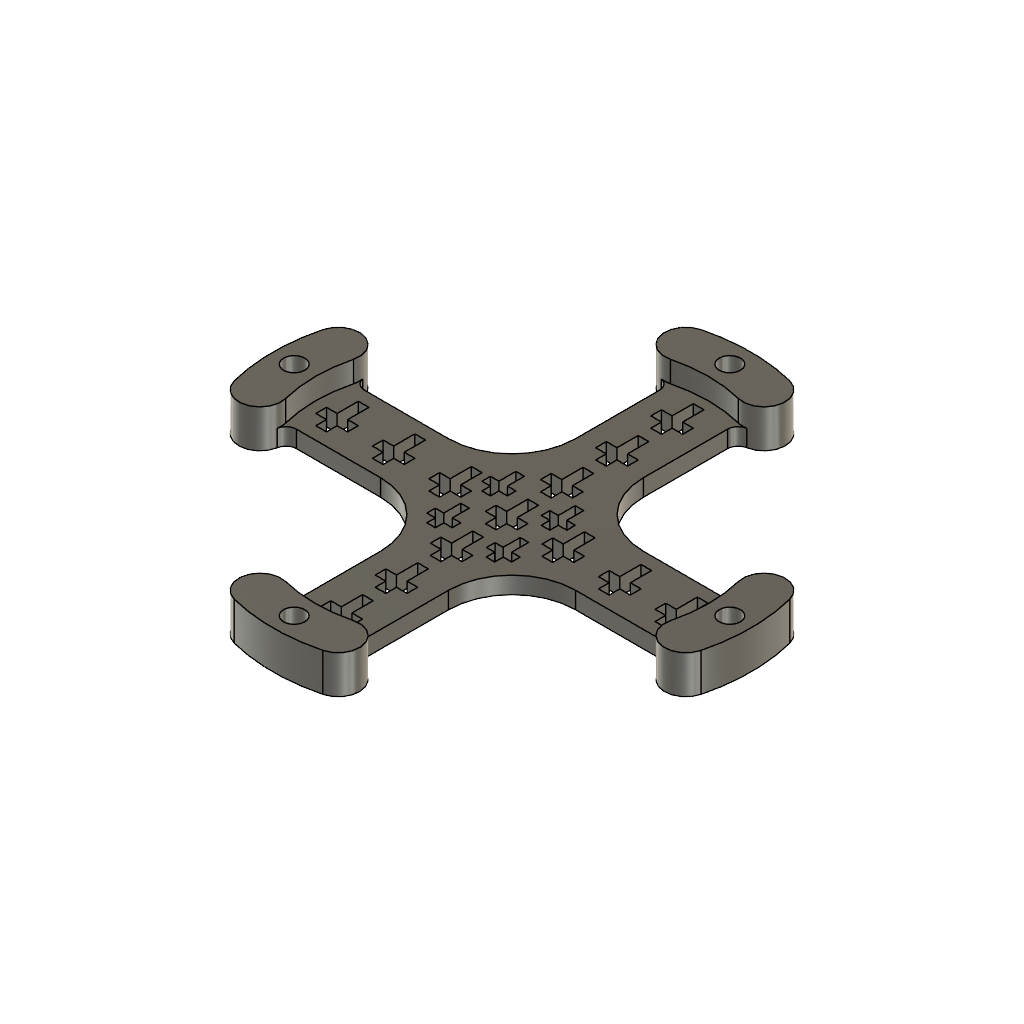
LR cross plus grill (Autodesk Fusion 360 design; units mm, degrees)
Autodesk Fusion 360 part; units mm, degrees
note: some values were not read from the file. Set by a fixed rule: which sketch regions a step uses.
(part 1 of 2)
sketch "Sketch1" plane through (0, 0, 0) normal (0, 0, 1) x (1, 0, 0)
  circle A0 centre (0, 0) radius 41.875
  line L0 (0, 41.875) -> (0, 45.375)
  line L1 (0, 45.375) -> (-8, 45.375)
  line L2 (0, 45.375) -> (8, 45.375)
  line L3 (0, 45.375) -> (0, 46.375)
  arc A1 (8, 45.375) -> (-8, 45.375) centre (0, 13.875) ccw
  arc A2 (10.4615, 55.0673) -> (-10.4615, 55.0673) centre (0, 13.875) ccw
  line L4 (-10.4615, 55.0673) -> (-8, 45.375)
  circle A3 centre (-9.2308, 50.2212) radius 5
  line L5 (0, 45.375) -> (0, 0)
  line L6 (-8, 45.375) -> (-8, 0)
  circle A4 centre (9.2308, 50.2212) radius 5
  line L7 (8, 45.375) -> (8, 0)
  line L8 (-45.375, 8) -> (0, 8)
  line L9 (-45.375, -8) -> (0, -8)
  circle A5 centre (-50.2212, -9.2308) radius 5
  arc A6 (-45.375, 8) -> (-45.375, -8) centre (-13.875, 0) ccw
  circle A7 centre (-50.2212, 9.2308) radius 5
  arc A8 (-55.0673, 10.4615) -> (-55.0673, -10.4615) centre (-13.875, 0) ccw
  line L10 (-8, -45.375) -> (-8, 0)
  line L11 (8, -45.375) -> (8, 0)
  circle A9 centre (9.2308, -50.2212) radius 5
  arc A10 (-8, -45.375) -> (8, -45.375) centre (0, -13.875) ccw
  circle A11 centre (-9.2308, -50.2212) radius 5
  arc A12 (-10.4615, -55.0673) -> (10.4615, -55.0673) centre (0, -13.875) ccw
  line L12 (45.375, -8) -> (0, -8)
  line L13 (45.375, 8) -> (0, 8)
  circle A13 centre (50.2212, 9.2308) radius 5
  arc A14 (45.375, -8) -> (45.375, 8) centre (13.875, 0) ccw
  circle A15 centre (50.2212, -9.2308) radius 5
  arc A16 (55.0673, -10.4615) -> (55.0673, 10.4615) centre (13.875, 0) ccw
  circle A17 centre (23, 23) radius 15
  circle A18 centre (-23, 23) radius 15
  circle A19 centre (-23, -23) radius 15
  circle A20 centre (23, -23) radius 15
  line L14 (0, 46.375) -> (0, 56.375)
  circle A21 centre (0, 51.375) radius 2.5
  circle A22 centre (-51.375, 0) radius 2.5
  circle A23 centre (0, -51.375) radius 2.5
  circle A24 centre (51.375, 0) radius 2.5
  arc A25 (-8, 42.8293) -> (-10.0769, 45.2933) centre (-10.5, 42.8293) ccw
  arc A26 (10.0769, 45.2933) -> (8, 42.8293) centre (10.5, 42.8293) ccw
  arc A27 (-42.8293, -8) -> (-45.2933, -10.0769) centre (-42.8293, -10.5) ccw
  arc A28 (-45.2933, 10.0769) -> (-42.8293, 8) centre (-42.8293, 10.5) ccw
  arc A29 (8, -42.8293) -> (10.0769, -45.2933) centre (10.5, -42.8293) ccw
  arc A30 (-10.0769, -45.2933) -> (-8, -42.8293) centre (-10.5, -42.8293) ccw
  arc A31 (42.8293, 8) -> (45.2933, 10.0769) centre (42.8293, 10.5) ccw
  arc A32 (45.2933, -10.0769) -> (42.8293, -8) centre (42.8293, -10.5) ccw
  dimension "d1" = 83.75
  dimension "d2" = 3.5
  dimension "d4" = 8
  dimension "d5" = 8
  dimension "d6" = 1
  dimension "d7" = 10
  dimension "d8" = 8
  dimension "d12" = 30
  dimension "d14" = 360
  dimension "d19" = 5
  dimension "d21" = 360
  dimension "d22" = 5
  dimension "d24" = 360
  constraint coincident A0.centre L5.end
  constraint coincident A0 L0.start
  constraint vertical L0
  constraint perpendicular L1 L3
  constraint coincident L3.end A1
  constraint midpoint L4 A3.centre
  constraint coincident A2.end A3
  constraint perpendicular L2 L5
  constraint symmetric A3 L5 A4
  constraint symmetric L5 L1.end L2.end
  constraint symmetric L5 L6.end L7.end
  constraint tangent L7 A17
  constraint tangent L13 A17
  constraint midpoint A2 L14.end
  constraint parallel L3 L14
  constraint midpoint L14 A21.centre
  constraint tangent A3 A25
  constraint tangent L6 A25
  constraint coincident A3 A25.end
  constraint coincident L6 A25.start
  constraint symmetric L5 A25.end A26.start
  constraint symmetric L5 A25 A26
  constraint symmetric L5 A25.start A26.end
  measures "d1" diameter of A0
  measures "d2" distance of L0.start L0.end
  measures "d4" distance of L0.end L1.end
  measures "d5" distance of L0.end L2.end
  measures "d6" distance of L0.end L3.end
  measures "d12" diameter of A17
  measures "d19" diameter of A21
  measures "d22" diameter of A25
extrude "Extrude1" add sketch "Sketch1" along normal blind 4 contours A0 L7 L11 L12 L13 | A0 L12 L13 A14 | L13 A13 A31 | L7 L13 A17 | L12 A15 A32 | L11 L12 A20 | A0 L5 L7 L13 | L6 L7 L8 L9 L10 L11 L12 L13 | A0 L9 L10 L11 L12 | A0 L0 L2 L5 L7 | A0 L5 L6 L8 | A0 L10 L11 A10 | A0 L0 L1 L5 L6 | A4 L7 A26 | L6 L8 A18 | A0 L6 L8 L9 L10 | L11 A9 A29 | L9 L10 A19 | L2 L3 A1 | L1 L3 A1 | L10 A11 A30 | A3 L6 A25 | A0 L8 L9 A6 | L8 A7 A28 | L9 A5 A27
extrude "Extrude2" add sketch "Sketch1" along normal blind 9 contours A13 | A13 A14 A15 A16 | A15 | A1 A2 A4 L14 A21 | A4 | A9 | A9 A10 A11 A12 | A1 A2 A3 L14 A21 | L4 A3 | L4 A3 | A11 | A5 A6 A7 A8 | A7 | A5
sketch "Sketch2" plane through (0, 0, 0) normal (0, 0, -1) x (1, 0, 0)
  circle A0 centre (0, 51.375) radius 2.5
  circle A1 centre (-51.375, 0) radius 2.5
  circle A2 centre (51.375, 0) radius 2.5
  circle A3 centre (0, -51.375) radius 2.5
  arc A4 (45.2933, -10.0769) -> (55.0673, -10.4615) centre (50.2212, -9.2308) ccw
  arc A5 (55.0673, -10.4615) -> (55.0673, 10.4615) centre (13.875, 0) ccw
  arc A6 (55.0673, 10.4615) -> (45.2933, 10.0769) centre (50.2212, 9.2308) ccw
  arc A7 (42.8293, 8) -> (45.2933, 10.0769) centre (42.8293, 10.5) ccw
  line L0 (42.8293, 8) -> (23, 8)
  arc A8 (8, 23) -> (23, 8) centre (23, 23) ccw
  line L1 (8, 23) -> (8, 42.8293)
  arc A9 (10.0769, 45.2933) -> (8, 42.8293) centre (10.5, 42.8293) ccw
  arc A10 (10.0769, 45.2933) -> (10.4615, 55.0673) centre (9.2308, 50.2212) ccw
  arc A11 (10.4615, 55.0673) -> (-10.4615, 55.0673) centre (0, 13.875) ccw
  arc A12 (-10.4615, 55.0673) -> (-10.0769, 45.2933) centre (-9.2308, 50.2212) ccw
  arc A13 (-8, 42.8293) -> (-10.0769, 45.2933) centre (-10.5, 42.8293) ccw
  line L2 (-8, 42.8293) -> (-8, 23)
  arc A14 (-23, 8) -> (-8, 23) centre (-23, 23) ccw
  line L3 (-23, 8) -> (-42.8293, 8)
  arc A15 (-45.2933, 10.0769) -> (-42.8293, 8) centre (-42.8293, 10.5) ccw
  arc A16 (-45.2933, 10.0769) -> (-55.0673, 10.4615) centre (-50.2212, 9.2308) ccw
  arc A17 (-55.0673, 10.4615) -> (-55.0673, -10.4615) centre (-13.875, 0) ccw
  arc A18 (-55.0673, -10.4615) -> (-45.2933, -10.0769) centre (-50.2212, -9.2308) ccw
  arc A19 (-42.8293, -8) -> (-45.2933, -10.0769) centre (-42.8293, -10.5) ccw
  line L4 (-42.8293, -8) -> (-23, -8)
  arc A20 (-8, -23) -> (-23, -8) centre (-23, -23) ccw
  line L5 (-8, -23) -> (-8, -42.8293)
  arc A21 (-10.0769, -45.2933) -> (-8, -42.8293) centre (-10.5, -42.8293) ccw
  arc A22 (-10.0769, -45.2933) -> (-10.4615, -55.0673) centre (-9.2308, -50.2212) ccw
  arc A23 (-10.4615, -55.0673) -> (10.4615, -55.0673) centre (0, -13.875) ccw
  arc A24 (10.4615, -55.0673) -> (10.0769, -45.2933) centre (9.2308, -50.2212) ccw
  arc A25 (8, -42.8293) -> (10.0769, -45.2933) centre (10.5, -42.8293) ccw
  line L6 (8, -42.8293) -> (8, -23)
  arc A26 (23, -8) -> (8, -23) centre (23, -23) ccw
  line L7 (23, -8) -> (42.8293, -8)
  arc A27 (45.2933, -10.0769) -> (42.8293, -8) centre (42.8293, -10.5) ccw
  line L8 (0, 0) -> (0, 5)
  line L9 (0, 5) -> (-1.25, 5)
  line L10 (-1.25, 5) -> (1.25, 5)
  line L11 (1.25, 5) -> (1.25, -5)
  line L12 (1.25, -5) -> (-1.25, -5)
  line L13 (-1.25, -5) -> (-1.25, 5)
  line L14 (-1.25, 5) -> (-1.25, 2.5)
  line L15 (-1.25, 2.5) -> (-3.75, 2.5)
  line L16 (-3.75, 2.5) -> (3.75, 2.5)
  line L17 (3.75, 2.5) -> (3.75, 0)
  line L18 (3.75, 0) -> (-3.75, 0)
  line L19 (-3.75, 0) -> (-3.75, 2.5)
  arc A28 (-8, -45.375) -> (8, -45.375) centre (0, -13.875) ccw
  arc A29 (-45.375, 8) -> (-45.375, -8) centre (-13.875, 0) ccw
  arc A30 (8, 45.375) -> (-8, 45.375) centre (0, 13.875) ccw
  arc A31 (45.375, -8) -> (45.375, 8) centre (13.875, 0) ccw
  line L20 (-38.75, -34) -> (-38.75, -44)
  line L21 (-41.25, -34) -> (-38.75, -34)
  line L22 (-41.25, -36.5) -> (-43.75, -36.5)
  line L23 (-41.25, -34) -> (-41.25, -36.5)
  line L24 (-43.75, -36.5) -> (-36.25, -36.5)
  line L25 (-40, -34) -> (-41.25, -34)
  line L26 (-40, -39) -> (-40, -34)
  line L27 (-41.25, -44) -> (-41.25, -34)
  line L28 (-43.75, -39) -> (-43.75, -36.5)
  line L29 (-38.75, -44) -> (-41.25, -44)
  line L30 (-36.25, -36.5) -> (-36.25, -39)
  line L31 (-36.25, -39) -> (-43.75, -39)
  line L32 (-25.4167, -34) -> (-25.4167, -44)
  line L33 (-27.9167, -34) -> (-25.4167, -34)
  line L34 (-27.9167, -36.5) -> (-30.4167, -36.5)
  line L35 (-27.9167, -34) -> (-27.9167, -36.5)
  line L36 (-30.4167, -36.5) -> (-22.9167, -36.5)
  line L37 (-26.6667, -34) -> (-27.9167, -34)
  line L38 (-26.6667, -39) -> (-26.6667, -34)
  line L39 (-27.9167, -44) -> (-27.9167, -34)
  line L40 (-30.4167, -39) -> (-30.4167, -36.5)
  line L41 (-25.4167, -44) -> (-27.9167, -44)
  line L42 (-22.9167, -36.5) -> (-22.9167, -39)
  line L43 (-22.9167, -39) -> (-30.4167, -39)
  line L44 (-12.0833, -34) -> (-12.0833, -44)
  line L45 (-14.5833, -34) -> (-12.0833, -34)
  line L46 (-14.5833, -36.5) -> (-17.0833, -36.5)
  line L47 (-14.5833, -34) -> (-14.5833, -36.5)
  line L48 (-17.0833, -36.5) -> (-9.5833, -36.5)
  line L49 (-13.3333, -34) -> (-14.5833, -34)
  line L50 (-13.3333, -39) -> (-13.3333, -34)
  line L51 (-14.5833, -44) -> (-14.5833, -34)
  line L52 (-17.0833, -39) -> (-17.0833, -36.5)
  line L53 (-12.0833, -44) -> (-14.5833, -44)
  line L54 (-9.5833, -36.5) -> (-9.5833, -39)
  line L55 (-9.5833, -39) -> (-17.0833, -39)
  line L56 (1.25, -34) -> (1.25, -44)
  line L57 (-1.25, -34) -> (1.25, -34)
  line L58 (-1.25, -36.5) -> (-3.75, -36.5)
  line L59 (-1.25, -34) -> (-1.25, -36.5)
  line L60 (-3.75, -36.5) -> (3.75, -36.5)
  line L61 (0, -34) -> (-1.25, -34)
  line L62 (0, -39) -> (0, -34)
  line L63 (-1.25, -44) -> (-1.25, -34)
  line L64 (-3.75, -39) -> (-3.75, -36.5)
  line L65 (1.25, -44) -> (-1.25, -44)
  line L66 (3.75, -36.5) -> (3.75, -39)
  line L67 (3.75, -39) -> (-3.75, -39)
  line L68 (14.5833, -34) -> (14.5833, -44)
  line L69 (12.0833, -34) -> (14.5833, -34)
  line L70 (12.0833, -36.5) -> (9.5833, -36.5)
  line L71 (12.0833, -34) -> (12.0833, -36.5)
  line L72 (9.5833, -36.5) -> (17.0833, -36.5)
  line L73 (13.3333, -34) -> (12.0833, -34)
  line L74 (13.3333, -39) -> (13.3333, -34)
  line L75 (12.0833, -44) -> (12.0833, -34)
  line L76 (9.5833, -39) -> (9.5833, -36.5)
  line L77 (14.5833, -44) -> (12.0833, -44)
  line L78 (17.0833, -36.5) -> (17.0833, -39)
  line L79 (17.0833, -39) -> (9.5833, -39)
  line L80 (27.9167, -34) -> (27.9167, -44)
  line L81 (25.4167, -34) -> (27.9167, -34)
  line L82 (25.4167, -36.5) -> (22.9167, -36.5)
  line L83 (25.4167, -34) -> (25.4167, -36.5)
  line L84 (22.9167, -36.5) -> (30.4167, -36.5)
  line L85 (26.6667, -34) -> (25.4167, -34)
  line L86 (26.6667, -39) -> (26.6667, -34)
  line L87 (25.4167, -44) -> (25.4167, -34)
  line L88 (22.9167, -39) -> (22.9167, -36.5)
  line L89 (27.9167, -44) -> (25.4167, -44)
  line L90 (30.4167, -36.5) -> (30.4167, -39)
  line L91 (30.4167, -39) -> (22.9167, -39)
  line L92 (41.25, -34) -> (41.25, -44)
  line L93 (38.75, -34) -> (41.25, -34)
  line L94 (38.75, -36.5) -> (36.25, -36.5)
  line L95 (38.75, -34) -> (38.75, -36.5)
  line L96 (36.25, -36.5) -> (43.75, -36.5)
  line L97 (40, -34) -> (38.75, -34)
  line L98 (40, -39) -> (40, -34)
  line L99 (38.75, -44) -> (38.75, -34)
  line L100 (36.25, -39) -> (36.25, -36.5)
  line L101 (41.25, -44) -> (38.75, -44)
  line L102 (43.75, -36.5) -> (43.75, -39)
  line L103 (43.75, -39) -> (36.25, -39)
  line L104 (-38.75, -21) -> (-38.75, -31)
  line L105 (-41.25, -21) -> (-38.75, -21)
  line L106 (-41.25, -23.5) -> (-43.75, -23.5)
  line L107 (-41.25, -21) -> (-41.25, -23.5)
  line L108 (-43.75, -23.5) -> (-36.25, -23.5)
  line L109 (-40, -21) -> (-41.25, -21)
  line L110 (-40, -26) -> (-40, -21)
  line L111 (-41.25, -31) -> (-41.25, -21)
  line L112 (-43.75, -26) -> (-43.75, -23.5)
  line L113 (-38.75, -31) -> (-41.25, -31)
  line L114 (-36.25, -23.5) -> (-36.25, -26)
  line L115 (-36.25, -26) -> (-43.75, -26)
  line L116 (-25.4167, -21) -> (-25.4167, -31)
  line L117 (-27.9167, -21) -> (-25.4167, -21)
  line L118 (-27.9167, -23.5) -> (-30.4167, -23.5)
  line L119 (-27.9167, -21) -> (-27.9167, -23.5)
  line L120 (-30.4167, -23.5) -> (-22.9167, -23.5)
  line L121 (-26.6667, -21) -> (-27.9167, -21)
  line L122 (-26.6667, -26) -> (-26.6667, -21)
  line L123 (-27.9167, -31) -> (-27.9167, -21)
  line L124 (-30.4167, -26) -> (-30.4167, -23.5)
  line L125 (-25.4167, -31) -> (-27.9167, -31)
  line L126 (-22.9167, -23.5) -> (-22.9167, -26)
  line L127 (-22.9167, -26) -> (-30.4167, -26)
  line L128 (-12.0833, -21) -> (-12.0833, -31)
  line L129 (-14.5833, -21) -> (-12.0833, -21)
  line L130 (-14.5833, -23.5) -> (-17.0833, -23.5)
  line L131 (-14.5833, -21) -> (-14.5833, -23.5)
  line L132 (-17.0833, -23.5) -> (-9.5833, -23.5)
  line L133 (-13.3333, -21) -> (-14.5833, -21)
  line L134 (-13.3333, -26) -> (-13.3333, -21)
  line L135 (-14.5833, -31) -> (-14.5833, -21)
  line L136 (-17.0833, -26) -> (-17.0833, -23.5)
  line L137 (-12.0833, -31) -> (-14.5833, -31)
  line L138 (-9.5833, -23.5) -> (-9.5833, -26)
  line L139 (-9.5833, -26) -> (-17.0833, -26)
  line L140 (1.25, -21) -> (1.25, -31)
  line L141 (-1.25, -21) -> (1.25, -21)
  line L142 (-1.25, -23.5) -> (-3.75, -23.5)
  line L143 (-1.25, -21) -> (-1.25, -23.5)
  line L144 (-3.75, -23.5) -> (3.75, -23.5)
  line L145 (0, -21) -> (-1.25, -21)
  line L146 (0, -26) -> (0, -21)
  line L147 (-1.25, -31) -> (-1.25, -21)
  line L148 (-3.75, -26) -> (-3.75, -23.5)
  line L149 (1.25, -31) -> (-1.25, -31)
  line L150 (3.75, -23.5) -> (3.75, -26)
  line L151 (3.75, -26) -> (-3.75, -26)
  line L152 (14.5833, -21) -> (14.5833, -31)
  line L153 (12.0833, -21) -> (14.5833, -21)
  line L154 (12.0833, -23.5) -> (9.5833, -23.5)
  line L155 (12.0833, -21) -> (12.0833, -23.5)
  line L156 (9.5833, -23.5) -> (17.0833, -23.5)
  line L157 (13.3333, -21) -> (12.0833, -21)
  line L158 (13.3333, -26) -> (13.3333, -21)
  line L159 (12.0833, -31) -> (12.0833, -21)
  line L160 (9.5833, -26) -> (9.5833, -23.5)
  line L161 (14.5833, -31) -> (12.0833, -31)
  line L162 (17.0833, -23.5) -> (17.0833, -26)
  line L163 (17.0833, -26) -> (9.5833, -26)
  line L164 (27.9167, -21) -> (27.9167, -31)
  line L165 (25.4167, -21) -> (27.9167, -21)
  line L166 (25.4167, -23.5) -> (22.9167, -23.5)
  line L167 (25.4167, -21) -> (25.4167, -23.5)
  line L168 (22.9167, -23.5) -> (30.4167, -23.5)
  line L169 (26.6667, -21) -> (25.4167, -21)
  line L170 (26.6667, -26) -> (26.6667, -21)
  line L171 (25.4167, -31) -> (25.4167, -21)
  line L172 (22.9167, -26) -> (22.9167, -23.5)
  line L173 (27.9167, -31) -> (25.4167, -31)
  line L174 (30.4167, -23.5) -> (30.4167, -26)
  line L175 (30.4167, -26) -> (22.9167, -26)
  line L176 (41.25, -21) -> (41.25, -31)
  line L177 (38.75, -21) -> (41.25, -21)
  line L178 (38.75, -23.5) -> (36.25, -23.5)
  line L179 (38.75, -21) -> (38.75, -23.5)
  line L180 (36.25, -23.5) -> (43.75, -23.5)
  line L181 (40, -21) -> (38.75, -21)
  line L182 (40, -26) -> (40, -21)
  line L183 (38.75, -31) -> (38.75, -21)
  line L184 (36.25, -26) -> (36.25, -23.5)
  line L185 (41.25, -31) -> (38.75, -31)
  line L186 (43.75, -23.5) -> (43.75, -26)
  line L187 (43.75, -26) -> (36.25, -26)
  line L188 (-38.75, -8) -> (-38.75, -18)
  line L189 (-41.25, -8) -> (-38.75, -8)
  line L190 (-41.25, -10.5) -> (-43.75, -10.5)
  line L191 (-41.25, -8) -> (-41.25, -10.5)
  line L192 (-43.75, -10.5) -> (-36.25, -10.5)
  line L193 (-40, -8) -> (-41.25, -8)
  line L194 (-40, -13) -> (-40, -8)
  line L195 (-41.25, -18) -> (-41.25, -8)
  line L196 (-43.75, -13) -> (-43.75, -10.5)
  line L197 (-38.75, -18) -> (-41.25, -18)
  line L198 (-36.25, -10.5) -> (-36.25, -13)
  line L199 (-36.25, -13) -> (-43.75, -13)
  line L200 (-25.4167, -8) -> (-25.4167, -18)
  line L201 (-27.9167, -8) -> (-25.4167, -8)
  line L202 (-27.9167, -10.5) -> (-30.4167, -10.5)
  line L203 (-27.9167, -8) -> (-27.9167, -10.5)
  line L204 (-30.4167, -10.5) -> (-22.9167, -10.5)
  line L205 (-26.6667, -8) -> (-27.9167, -8)
  line L206 (-26.6667, -13) -> (-26.6667, -8)
  line L207 (-27.9167, -18) -> (-27.9167, -8)
  line L208 (-30.4167, -13) -> (-30.4167, -10.5)
  line L209 (-25.4167, -18) -> (-27.9167, -18)
  line L210 (-22.9167, -10.5) -> (-22.9167, -13)
  line L211 (-22.9167, -13) -> (-30.4167, -13)
  line L212 (-12.0833, -8) -> (-12.0833, -18)
  line L213 (-14.5833, -8) -> (-12.0833, -8)
  line L214 (-14.5833, -10.5) -> (-17.0833, -10.5)
  line L215 (-14.5833, -8) -> (-14.5833, -10.5)
  line L216 (-17.0833, -10.5) -> (-9.5833, -10.5)
  line L217 (-13.3333, -8) -> (-14.5833, -8)
  line L218 (-13.3333, -13) -> (-13.3333, -8)
  line L219 (-14.5833, -18) -> (-14.5833, -8)
  line L220 (-17.0833, -13) -> (-17.0833, -10.5)
  line L221 (-12.0833, -18) -> (-14.5833, -18)
  line L222 (-9.5833, -10.5) -> (-9.5833, -13)
  line L223 (-9.5833, -13) -> (-17.0833, -13)
  line L224 (1.25, -8) -> (1.25, -18)
  line L225 (-1.25, -8) -> (1.25, -8)
  line L226 (-1.25, -10.5) -> (-3.75, -10.5)
  line L227 (-1.25, -8) -> (-1.25, -10.5)
  line L228 (-3.75, -10.5) -> (3.75, -10.5)
  line L229 (0, -8) -> (-1.25, -8)
  line L230 (0, -13) -> (0, -8)
  line L231 (-1.25, -18) -> (-1.25, -8)
  line L232 (-3.75, -13) -> (-3.75, -10.5)
  line L233 (1.25, -18) -> (-1.25, -18)
  line L234 (3.75, -10.5) -> (3.75, -13)
  line L235 (3.75, -13) -> (-3.75, -13)
  line L236 (14.5833, -8) -> (14.5833, -18)
  line L237 (12.0833, -8) -> (14.5833, -8)
  line L238 (12.0833, -10.5) -> (9.5833, -10.5)
  line L239 (12.0833, -8) -> (12.0833, -10.5)
  line L240 (9.5833, -10.5) -> (17.0833, -10.5)
  line L241 (13.3333, -8) -> (12.0833, -8)
  line L242 (13.3333, -13) -> (13.3333, -8)
  line L243 (12.0833, -18) -> (12.0833, -8)
  line L244 (9.5833, -13) -> (9.5833, -10.5)
  line L245 (14.5833, -18) -> (12.0833, -18)
  line L246 (17.0833, -10.5) -> (17.0833, -13)
  line L247 (17.0833, -13) -> (9.5833, -13)
  line L248 (27.9167, -8) -> (27.9167, -18)
  line L249 (25.4167, -8) -> (27.9167, -8)
  line L250 (25.4167, -10.5) -> (22.9167, -10.5)
  line L251 (25.4167, -8) -> (25.4167, -10.5)
  line L252 (22.9167, -10.5) -> (30.4167, -10.5)
  line L253 (26.6667, -8) -> (25.4167, -8)
  line L254 (26.6667, -13) -> (26.6667, -8)
  line L255 (25.4167, -18) -> (25.4167, -8)
  line L256 (22.9167, -13) -> (22.9167, -10.5)
  line L257 (27.9167, -18) -> (25.4167, -18)
  line L258 (30.4167, -10.5) -> (30.4167, -13)
  line L259 (30.4167, -13) -> (22.9167, -13)
  line L260 (41.25, -8) -> (41.25, -18)
  line L261 (38.75, -8) -> (41.25, -8)
  line L262 (38.75, -10.5) -> (36.25, -10.5)
  line L263 (38.75, -8) -> (38.75, -10.5)
  line L264 (36.25, -10.5) -> (43.75, -10.5)
  line L265 (40, -8) -> (38.75, -8)
  line L266 (40, -13) -> (40, -8)
  line L267 (38.75, -18) -> (38.75, -8)
  line L268 (36.25, -13) -> (36.25, -10.5)
  line L269 (41.25, -18) -> (38.75, -18)
  line L270 (43.75, -10.5) -> (43.75, -13)
  line L271 (43.75, -13) -> (36.25, -13)
  line L272 (-38.75, 5) -> (-38.75, -5)
  line L273 (-41.25, 5) -> (-38.75, 5)
  line L274 (-41.25, 2.5) -> (-43.75, 2.5)
  line L275 (-41.25, 5) -> (-41.25, 2.5)
  line L276 (-43.75, 2.5) -> (-36.25, 2.5)
  line L277 (-40, 5) -> (-41.25, 5)
  line L278 (-40, 0) -> (-40, 5)
  line L279 (-41.25, -5) -> (-41.25, 5)
  line L280 (-43.75, 0) -> (-43.75, 2.5)
  line L281 (-38.75, -5) -> (-41.25, -5)
  line L282 (-36.25, 2.5) -> (-36.25, 0)
  line L283 (-36.25, 0) -> (-43.75, 0)
  line L284 (-25.4167, 5) -> (-25.4167, -5)
  line L285 (-27.9167, 5) -> (-25.4167, 5)
  line L286 (-27.9167, 2.5) -> (-30.4167, 2.5)
  line L287 (-27.9167, 5) -> (-27.9167, 2.5)
  line L288 (-30.4167, 2.5) -> (-22.9167, 2.5)
  line L289 (-26.6667, 5) -> (-27.9167, 5)
  line L290 (-26.6667, 0) -> (-26.6667, 5)
  line L291 (-27.9167, -5) -> (-27.9167, 5)
  line L292 (-30.4167, 0) -> (-30.4167, 2.5)
  line L293 (-25.4167, -5) -> (-27.9167, -5)
  line L294 (-22.9167, 2.5) -> (-22.9167, 0)
  line L295 (-22.9167, 0) -> (-30.4167, 0)
  line L296 (-12.0833, 5) -> (-12.0833, -5)
  line L297 (-14.5833, 5) -> (-12.0833, 5)
  line L298 (-14.5833, 2.5) -> (-17.0833, 2.5)
  line L299 (-14.5833, 5) -> (-14.5833, 2.5)
  line L300 (-17.0833, 2.5) -> (-9.5833, 2.5)
  line L301 (-13.3333, 5) -> (-14.5833, 5)
  line L302 (-13.3333, 0) -> (-13.3333, 5)
  line L303 (-14.5833, -5) -> (-14.5833, 5)
  line L304 (-17.0833, 0) -> (-17.0833, 2.5)
  line L305 (-12.0833, -5) -> (-14.5833, -5)
  line L306 (-9.5833, 2.5) -> (-9.5833, 0)
  line L307 (-9.5833, 0) -> (-17.0833, 0)
  line L308 (14.5833, 5) -> (14.5833, -5)
  line L309 (12.0833, 5) -> (14.5833, 5)
  line L310 (12.0833, 2.5) -> (9.5833, 2.5)
  line L311 (12.0833, 5) -> (12.0833, 2.5)
  line L312 (9.5833, 2.5) -> (17.0833, 2.5)
  line L313 (13.3333, 5) -> (12.0833, 5)
  line L314 (13.3333, 0) -> (13.3333, 5)
  line L315 (12.0833, -5) -> (12.0833, 5)
  line L316 (9.5833, 0) -> (9.5833, 2.5)
  line L317 (14.5833, -5) -> (12.0833, -5)
  line L318 (17.0833, 2.5) -> (17.0833, 0)
  line L319 (17.0833, 0) -> (9.5833, 0)
  line L320 (27.9167, 5) -> (27.9167, -5)
  line L321 (25.4167, 5) -> (27.9167, 5)
  line L322 (25.4167, 2.5) -> (22.9167, 2.5)
  line L323 (25.4167, 5) -> (25.4167, 2.5)
  line L324 (22.9167, 2.5) -> (30.4167, 2.5)
  line L325 (26.6667, 5) -> (25.4167, 5)
  line L326 (26.6667, 0) -> (26.6667, 5)
  line L327 (25.4167, -5) -> (25.4167, 5)
  line L328 (22.9167, 0) -> (22.9167, 2.5)
  line L329 (27.9167, -5) -> (25.4167, -5)
  line L330 (30.4167, 2.5) -> (30.4167, 0)
  line L331 (30.4167, 0) -> (22.9167, 0)
  line L332 (41.25, 5) -> (41.25, -5)
  line L333 (38.75, 5) -> (41.25, 5)
  line L334 (38.75, 2.5) -> (36.25, 2.5)
  line L335 (38.75, 5) -> (38.75, 2.5)
  line L336 (36.25, 2.5) -> (43.75, 2.5)
  line L337 (40, 5) -> (38.75, 5)
  line L338 (40, 0) -> (40, 5)
  line L339 (38.75, -5) -> (38.75, 5)
  line L340 (36.25, 0) -> (36.25, 2.5)
  line L341 (41.25, -5) -> (38.75, -5)
  line L342 (43.75, 2.5) -> (43.75, 0)
  line L343 (43.75, 0) -> (36.25, 0)
  line L344 (-38.75, 18) -> (-38.75, 8)
  line L345 (-41.25, 18) -> (-38.75, 18)
  line L346 (-41.25, 15.5) -> (-43.75, 15.5)
  line L347 (-41.25, 18) -> (-41.25, 15.5)
  line L348 (-43.75, 15.5) -> (-36.25, 15.5)
  line L349 (-40, 18) -> (-41.25, 18)
  line L350 (-40, 13) -> (-40, 18)
  line L351 (-41.25, 8) -> (-41.25, 18)
  line L352 (-43.75, 13) -> (-43.75, 15.5)
  line L353 (-38.75, 8) -> (-41.25, 8)
  line L354 (-36.25, 15.5) -> (-36.25, 13)
  line L355 (-36.25, 13) -> (-43.75, 13)
  line L356 (-25.4167, 18) -> (-25.4167, 8)
  line L357 (-27.9167, 18) -> (-25.4167, 18)
  line L358 (-27.9167, 15.5) -> (-30.4167, 15.5)
  line L359 (-27.9167, 18) -> (-27.9167, 15.5)
  line L360 (-30.4167, 15.5) -> (-22.9167, 15.5)
  line L361 (-26.6667, 18) -> (-27.9167, 18)
  line L362 (-26.6667, 13) -> (-26.6667, 18)
  line L363 (-27.9167, 8) -> (-27.9167, 18)
  line L364 (-30.4167, 13) -> (-30.4167, 15.5)
  line L365 (-25.4167, 8) -> (-27.9167, 8)
  line L366 (-22.9167, 15.5) -> (-22.9167, 13)
  line L367 (-22.9167, 13) -> (-30.4167, 13)
  line L368 (-12.0833, 18) -> (-12.0833, 8)
  line L369 (-14.5833, 18) -> (-12.0833, 18)
  line L370 (-14.5833, 15.5) -> (-17.0833, 15.5)
  line L371 (-14.5833, 18) -> (-14.5833, 15.5)
  line L372 (-17.0833, 15.5) -> (-9.5833, 15.5)
  line L373 (-13.3333, 18) -> (-14.5833, 18)
  line L374 (-13.3333, 13) -> (-13.3333, 18)
  line L375 (-14.5833, 8) -> (-14.5833, 18)
  line L376 (-17.0833, 13) -> (-17.0833, 15.5)
  line L377 (-12.0833, 8) -> (-14.5833, 8)
  line L378 (-9.5833, 15.5) -> (-9.5833, 13)
  line L379 (-9.5833, 13) -> (-17.0833, 13)
  line L380 (1.25, 18) -> (1.25, 8)
  line L381 (-1.25, 18) -> (1.25, 18)
  line L382 (-1.25, 15.5) -> (-3.75, 15.5)
  line L383 (-1.25, 18) -> (-1.25, 15.5)
  line L384 (-3.75, 15.5) -> (3.75, 15.5)
  line L385 (0, 18) -> (-1.25, 18)
  line L386 (0, 13) -> (0, 18)
  line L387 (-1.25, 8) -> (-1.25, 18)
  line L388 (-3.75, 13) -> (-3.75, 15.5)
  line L389 (1.25, 8) -> (-1.25, 8)
  line L390 (3.75, 15.5) -> (3.75, 13)
  line L391 (3.75, 13) -> (-3.75, 13)
  line L392 (14.5833, 18) -> (14.5833, 8)
  line L393 (12.0833, 18) -> (14.5833, 18)
  line L394 (12.0833, 15.5) -> (9.5833, 15.5)
  line L395 (12.0833, 18) -> (12.0833, 15.5)
  line L396 (9.5833, 15.5) -> (17.0833, 15.5)
  line L397 (13.3333, 18) -> (12.0833, 18)
  line L398 (13.3333, 13) -> (13.3333, 18)
  line L399 (12.0833, 8) -> (12.0833, 18)
  line L400 (9.5833, 13) -> (9.5833, 15.5)
  line L401 (14.5833, 8) -> (12.0833, 8)
  line L402 (17.0833, 15.5) -> (17.0833, 13)
  line L403 (17.0833, 13) -> (9.5833, 13)
  line L404 (27.9167, 18) -> (27.9167, 8)
  line L405 (25.4167, 18) -> (27.9167, 18)
  line L406 (25.4167, 15.5) -> (22.9167, 15.5)
  line L407 (25.4167, 18) -> (25.4167, 15.5)
  line L408 (22.9167, 15.5) -> (30.4167, 15.5)
  line L409 (26.6667, 18) -> (25.4167, 18)
  line L410 (26.6667, 13) -> (26.6667, 18)
  line L411 (25.4167, 8) -> (25.4167, 18)
  line L412 (22.9167, 13) -> (22.9167, 15.5)
  line L413 (27.9167, 8) -> (25.4167, 8)
  line L414 (30.4167, 15.5) -> (30.4167, 13)
  line L415 (30.4167, 13) -> (22.9167, 13)
  line L416 (41.25, 18) -> (41.25, 8)
  line L417 (38.75, 18) -> (41.25, 18)
  line L418 (38.75, 15.5) -> (36.25, 15.5)
  line L419 (38.75, 18) -> (38.75, 15.5)
  line L420 (36.25, 15.5) -> (43.75, 15.5)
  line L421 (40, 18) -> (38.75, 18)
  line L422 (40, 13) -> (40, 18)
  line L423 (38.75, 8) -> (38.75, 18)
  line L424 (36.25, 13) -> (36.25, 15.5)
  line L425 (41.25, 8) -> (38.75, 8)
  line L426 (43.75, 15.5) -> (43.75, 13)
  line L427 (43.75, 13) -> (36.25, 13)
  line L428 (-38.75, 31) -> (-38.75, 21)
  line L429 (-41.25, 31) -> (-38.75, 31)
  line L430 (-41.25, 28.5) -> (-43.75, 28.5)
  line L431 (-41.25, 31) -> (-41.25, 28.5)
  line L432 (-43.75, 28.5) -> (-36.25, 28.5)
  line L433 (-40, 31) -> (-41.25, 31)
  line L434 (-40, 26) -> (-40, 31)
  line L435 (-41.25, 21) -> (-41.25, 31)
  line L436 (-43.75, 26) -> (-43.75, 28.5)
  line L437 (-38.75, 21) -> (-41.25, 21)
  line L438 (-36.25, 28.5) -> (-36.25, 26)
  line L439 (-36.25, 26) -> (-43.75, 26)
  line L440 (-25.4167, 31) -> (-25.4167, 21)
  line L441 (-27.9167, 31) -> (-25.4167, 31)
  line L442 (-27.9167, 28.5) -> (-30.4167, 28.5)
  line L443 (-27.9167, 31) -> (-27.9167, 28.5)
  line L444 (-30.4167, 28.5) -> (-22.9167, 28.5)
  line L445 (-26.6667, 31) -> (-27.9167, 31)
  line L446 (-26.6667, 26) -> (-26.6667, 31)
  line L447 (-27.9167, 21) -> (-27.9167, 31)
  line L448 (-30.4167, 26) -> (-30.4167, 28.5)
  line L449 (-25.4167, 21) -> (-27.9167, 21)
  line L450 (-22.9167, 28.5) -> (-22.9167, 26)
  line L451 (-22.9167, 26) -> (-30.4167, 26)
  line L452 (-12.0833, 31) -> (-12.0833, 21)
  line L453 (-14.5833, 31) -> (-12.0833, 31)
  line L454 (-14.5833, 28.5) -> (-17.0833, 28.5)
  line L455 (-14.5833, 31) -> (-14.5833, 28.5)
  line L456 (-17.0833, 28.5) -> (-9.5833, 28.5)
  line L457 (-13.3333, 31) -> (-14.5833, 31)
  line L458 (-13.3333, 26) -> (-13.3333, 31)
  line L459 (-14.5833, 21) -> (-14.5833, 31)
  line L460 (-17.0833, 26) -> (-17.0833, 28.5)
  line L461 (-12.0833, 21) -> (-14.5833, 21)
  line L462 (-9.5833, 28.5) -> (-9.5833, 26)
  line L463 (-9.5833, 26) -> (-17.0833, 26)
  line L464 (1.25, 31) -> (1.25, 21)
  line L465 (-1.25, 31) -> (1.25, 31)
  line L466 (-1.25, 28.5) -> (-3.75, 28.5)
  line L467 (-1.25, 31) -> (-1.25, 28.5)
  line L468 (-3.75, 28.5) -> (3.75, 28.5)
  line L469 (0, 31) -> (-1.25, 31)
  line L470 (0, 26) -> (0, 31)
  line L471 (-1.25, 21) -> (-1.25, 31)
  line L472 (-3.75, 26) -> (-3.75, 28.5)
  line L473 (1.25, 21) -> (-1.25, 21)
  line L474 (3.75, 28.5) -> (3.75, 26)
  line L475 (3.75, 26) -> (-3.75, 26)
  line L476 (14.5833, 31) -> (14.5833, 21)
  line L477 (12.0833, 31) -> (14.5833, 31)
  line L478 (12.0833, 28.5) -> (9.5833, 28.5)
  line L479 (12.0833, 31) -> (12.0833, 28.5)
  line L480 (9.5833, 28.5) -> (17.0833, 28.5)
  line L481 (13.3333, 31) -> (12.0833, 31)
  line L482 (13.3333, 26) -> (13.3333, 31)
  line L483 (12.0833, 21) -> (12.0833, 31)
  line L484 (9.5833, 26) -> (9.5833, 28.5)
  line L485 (14.5833, 21) -> (12.0833, 21)
  line L486 (17.0833, 28.5) -> (17.0833, 26)
  line L487 (17.0833, 26) -> (9.5833, 26)
  line L488 (27.9167, 31) -> (27.9167, 21)
  line L489 (25.4167, 31) -> (27.9167, 31)
  line L490 (25.4167, 28.5) -> (22.9167, 28.5)
  line L491 (25.4167, 31) -> (25.4167, 28.5)
  line L492 (22.9167, 28.5) -> (30.4167, 28.5)
  line L493 (26.6667, 31) -> (25.4167, 31)
  line L494 (26.6667, 26) -> (26.6667, 31)
  line L495 (25.4167, 21) -> (25.4167, 31)
  line L496 (22.9167, 26) -> (22.9167, 28.5)
  line L497 (27.9167, 21) -> (25.4167, 21)
  line L498 (30.4167, 28.5) -> (30.4167, 26)
  line L499 (30.4167, 26) -> (22.9167, 26)
  line L500 (41.25, 31) -> (41.25, 21)
  line L501 (38.75, 31) -> (41.25, 31)
  line L502 (38.75, 28.5) -> (36.25, 28.5)
  line L503 (38.75, 31) -> (38.75, 28.5)
  line L504 (36.25, 28.5) -> (43.75, 28.5)
  line L505 (40, 31) -> (38.75, 31)
  line L506 (40, 26) -> (40, 31)
  line L507 (38.75, 21) -> (38.75, 31)
  line L508 (36.25, 26) -> (36.25, 28.5)
  line L509 (41.25, 21) -> (38.75, 21)
  line L510 (43.75, 28.5) -> (43.75, 26)
  line L511 (43.75, 26) -> (36.25, 26)
  line L512 (-38.75, 44) -> (-38.75, 34)
  line L513 (-41.25, 44) -> (-38.75, 44)
  line L514 (-41.25, 41.5) -> (-43.75, 41.5)
  line L515 (-41.25, 44) -> (-41.25, 41.5)
  line L516 (-43.75, 41.5) -> (-36.25, 41.5)
  line L517 (-40, 44) -> (-41.25, 44)
  line L518 (-40, 39) -> (-40, 44)
  line L519 (-41.25, 34) -> (-41.25, 44)
  line L520 (-43.75, 39) -> (-43.75, 41.5)
  line L521 (-38.75, 34) -> (-41.25, 34)
  line L522 (-36.25, 41.5) -> (-36.25, 39)
  line L523 (-36.25, 39) -> (-43.75, 39)
  line L524 (-25.4167, 44) -> (-25.4167, 34)
  line L525 (-27.9167, 44) -> (-25.4167, 44)
  line L526 (-27.9167, 41.5) -> (-30.4167, 41.5)
  line L527 (-27.9167, 44) -> (-27.9167, 41.5)
  line L528 (-30.4167, 41.5) -> (-22.9167, 41.5)
  line L529 (-26.6667, 44) -> (-27.9167, 44)
  line L530 (-26.6667, 39) -> (-26.6667, 44)
  line L531 (-27.9167, 34) -> (-27.9167, 44)
  line L532 (-30.4167, 39) -> (-30.4167, 41.5)
  line L533 (-25.4167, 34) -> (-27.9167, 34)
  line L534 (-22.9167, 41.5) -> (-22.9167, 39)
  line L535 (-22.9167, 39) -> (-30.4167, 39)
  line L536 (-12.0833, 44) -> (-12.0833, 34)
  line L537 (-14.5833, 44) -> (-12.0833, 44)
  line L538 (-14.5833, 41.5) -> (-17.0833, 41.5)
  line L539 (-14.5833, 44) -> (-14.5833, 41.5)
  line L540 (-17.0833, 41.5) -> (-9.5833, 41.5)
  line L541 (-13.3333, 44) -> (-14.5833, 44)
  line L542 (-13.3333, 39) -> (-13.3333, 44)
  line L543 (-14.5833, 34) -> (-14.5833, 44)
  line L544 (-17.0833, 39) -> (-17.0833, 41.5)
  line L545 (-12.0833, 34) -> (-14.5833, 34)
  line L546 (-9.5833, 41.5) -> (-9.5833, 39)
  line L547 (-9.5833, 39) -> (-17.0833, 39)
  line L548 (1.25, 44) -> (1.25, 34)
  line L549 (-1.25, 44) -> (1.25, 44)
  line L550 (-1.25, 41.5) -> (-3.75, 41.5)
  line L551 (-1.25, 44) -> (-1.25, 41.5)
  line L552 (-3.75, 41.5) -> (3.75, 41.5)
  line L553 (0, 44) -> (-1.25, 44)
  line L554 (0, 39) -> (0, 44)
  line L555 (-1.25, 34) -> (-1.25, 44)
  line L556 (-3.75, 39) -> (-3.75, 41.5)
  line L557 (1.25, 34) -> (-1.25, 34)
  line L558 (3.75, 41.5) -> (3.75, 39)
  line L559 (3.75, 39) -> (-3.75, 39)
  line L560 (14.5833, 44) -> (14.5833, 34)
  line L561 (12.0833, 44) -> (14.5833, 44)
  line L562 (12.0833, 41.5) -> (9.5833, 41.5)
  line L563 (12.0833, 44) -> (12.0833, 41.5)
  line L564 (9.5833, 41.5) -> (17.0833, 41.5)
  line L565 (13.3333, 44) -> (12.0833, 44)
  line L566 (13.3333, 39) -> (13.3333, 44)
  line L567 (12.0833, 34) -> (12.0833, 44)
  line L568 (9.5833, 39) -> (9.5833, 41.5)
  line L569 (14.5833, 34) -> (12.0833, 34)
  line L570 (17.0833, 41.5) -> (17.0833, 39)
  line L571 (17.0833, 39) -> (9.5833, 39)
  line L572 (27.9167, 44) -> (27.9167, 34)
  line L573 (25.4167, 44) -> (27.9167, 44)
  line L574 (25.4167, 41.5) -> (22.9167, 41.5)
  line L575 (25.4167, 44) -> (25.4167, 41.5)
  line L576 (22.9167, 41.5) -> (30.4167, 41.5)
  line L577 (26.6667, 44) -> (25.4167, 44)
  line L578 (26.6667, 39) -> (26.6667, 44)
  line L579 (25.4167, 34) -> (25.4167, 44)
  line L580 (22.9167, 39) -> (22.9167, 41.5)
  line L581 (27.9167, 34) -> (25.4167, 34)
  line L582 (30.4167, 41.5) -> (30.4167, 39)
  line L583 (30.4167, 39) -> (22.9167, 39)
  line L584 (41.25, 44) -> (41.25, 34)
  line L585 (38.75, 44) -> (41.25, 44)
  line L586 (38.75, 41.5) -> (36.25, 41.5)
  line L587 (38.75, 44) -> (38.75, 41.5)
  line L588 (36.25, 41.5) -> (43.75, 41.5)
  line L589 (40, 44) -> (38.75, 44)
  line L590 (40, 39) -> (40, 44)
  line L591 (38.75, 34) -> (38.75, 44)
  line L592 (36.25, 39) -> (36.25, 41.5)
  line L593 (41.25, 34) -> (38.75, 34)
  line L594 (43.75, 41.5) -> (43.75, 39)
  line L595 (43.75, 39) -> (36.25, 39)
  line L596 (3.75, 2.5) -> (3.75, 13)
  line L597 (3.75, 2.5) -> (9.5833, 2.5)
  line L598 (3.75, 7.75) -> (6.6667, 7.75)
  line L599 (6.6667, 7.75) -> (6.6667, 11.75)
  line L600 (6.6667, 11.75) -> (5.6667, 11.75)
  line L601 (5.6667, 11.75) -> (7.6667, 11.75)
  line L602 (7.6667, 11.75) -> (7.6667, 3.75)
  line L603 (7.6667, 3.75) -> (5.6667, 3.75)
  line L604 (5.6667, 3.75) -> (5.6667, 11.75)
  line L605 (5.6667, 11.75) -> (5.6667, 9.75)
  line L606 (5.6667, 9.75) -> (3.6667, 9.75)
  line L607 (3.6667, 9.75) -> (9.6667, 9.75)
  line L608 (9.6667, 9.75) -> (9.6667, 7.75)
  line L609 (9.6667, 7.75) -> (3.6667, 7.75)
  line L610 (3.6667, 7.75) -> (3.6667, 9.75)
  line L611 (-8.3333, 9.75) -> (-10.3333, 9.75)
  line L612 (-4.3333, 7.75) -> (-10.3333, 7.75)
  line L613 (-8.3333, 11.75) -> (-8.3333, 9.75)
  line L614 (-7.3333, 7.75) -> (-7.3333, 11.75)
  line L615 (-10.25, 7.75) -> (-7.3333, 7.75)
  line L616 (-10.3333, 7.75) -> (-10.3333, 9.75)
  line L617 (-10.3333, 9.75) -> (-4.3333, 9.75)
  line L618 (-7.3333, 11.75) -> (-8.3333, 11.75)
  line L619 (-6.3333, 3.75) -> (-8.3333, 3.75)
  line L620 (-6.3333, 11.75) -> (-6.3333, 3.75)
  line L621 (-4.3333, 9.75) -> (-4.3333, 7.75)
  line L622 (-8.3333, 11.75) -> (-6.3333, 11.75)
  line L623 (-8.3333, 3.75) -> (-8.3333, 11.75)
  line L624 (5.6667, -3.25) -> (3.6667, -3.25)
  line L625 (9.6667, -5.25) -> (3.6667, -5.25)
  line L626 (5.6667, -1.25) -> (5.6667, -3.25)
  line L627 (6.6667, -5.25) -> (6.6667, -1.25)
  line L628 (3.75, -5.25) -> (6.6667, -5.25)
  line L629 (3.6667, -5.25) -> (3.6667, -3.25)
  line L630 (3.6667, -3.25) -> (9.6667, -3.25)
  line L631 (6.6667, -1.25) -> (5.6667, -1.25)
  line L632 (7.6667, -9.25) -> (5.6667, -9.25)
  line L633 (7.6667, -1.25) -> (7.6667, -9.25)
  line L634 (9.6667, -3.25) -> (9.6667, -5.25)
  line L635 (5.6667, -1.25) -> (7.6667, -1.25)
  line L636 (5.6667, -9.25) -> (5.6667, -1.25)
  line L637 (-8.3333, -3.25) -> (-10.3333, -3.25)
  line L638 (-4.3333, -5.25) -> (-10.3333, -5.25)
  line L639 (-8.3333, -1.25) -> (-8.3333, -3.25)
  line L640 (-7.3333, -5.25) -> (-7.3333, -1.25)
  line L641 (-10.25, -5.25) -> (-7.3333, -5.25)
  line L642 (-10.3333, -5.25) -> (-10.3333, -3.25)
  line L643 (-10.3333, -3.25) -> (-4.3333, -3.25)
  line L644 (-7.3333, -1.25) -> (-8.3333, -1.25)
  line L645 (-6.3333, -9.25) -> (-8.3333, -9.25)
  line L646 (-6.3333, -1.25) -> (-6.3333, -9.25)
  line L647 (-4.3333, -3.25) -> (-4.3333, -5.25)
  line L648 (-8.3333, -1.25) -> (-6.3333, -1.25)
  line L649 (-8.3333, -9.25) -> (-8.3333, -1.25)
  point P0 (-40, -39)
  point P1 (-26.6667, -39)
  point P2 (-13.3333, -39)
  point P3 (0, -39)
  point P4 (13.3333, -39)
  point P5 (26.6667, -39)
  point P6 (40, -39)
  point P7 (-40, -26)
  point P8 (-26.6667, -26)
  point P9 (-13.3333, -26)
  point P10 (0, -26)
  point P11 (13.3333, -26)
  point P12 (26.6667, -26)
  point P13 (40, -26)
  point P14 (-40, -13)
  point P15 (-26.6667, -13)
  point P16 (-13.3333, -13)
  point P17 (0, -13)
  point P18 (13.3333, -13)
  point P19 (26.6667, -13)
  point P20 (40, -13)
  point P21 (-40, 0)
  point P22 (-26.6667, 0)
  point P23 (-13.3333, 0)
  point P24 (13.3333, 0)
  point P25 (26.6667, 0)
  point P26 (40, 0)
  point P27 (-40, 13)
  point P28 (-26.6667, 13)
  point P29 (-13.3333, 13)
  point P30 (0, 13)
  point P31 (13.3333, 13)
  point P32 (26.6667, 13)
  point P33 (40, 13)
  point P34 (-40, 26)
  point P35 (-26.6667, 26)
  point P36 (-13.3333, 26)
  point P37 (0, 26)
  point P38 (13.3333, 26)
  point P39 (26.6667, 26)
  point P40 (40, 26)
  point P41 (-40, 39)
  point P42 (-26.6667, 39)
  point P43 (-13.3333, 39)
  point P44 (0, 39)
  point P45 (13.3333, 39)
  point P46 (26.6667, 39)
  point P47 (40, 39)
  dimension "d25" = 5
  dimension "d26" = 1.25
  dimension "d27" = 2.5
  dimension "d28" = 10
  dimension "d29" = 2.5
  dimension "d30" = 2.5
  dimension "d31" = 7.5
  dimension "d32" = 2.5
  dimension "d35" = 40
  dimension "d36" = 39
  dimension "d37" = 4
  dimension "d38" = 1
  dimension "d39" = 2
  dimension "d40" = 8
  dimension "d41" = 2
  dimension "d42" = 2
  dimension "d43" = 6
  dimension "d44" = 2
  dimension "d47" = -14
  dimension "d48" = -13
  constraint coincident L8.start origin
  constraint vertical L8
  constraint perpendicular L8 L9
  constraint horizontal L10
  constraint vertical L11
  constraint horizontal L12
  constraint vertical L13
  constraint perpendicular L9 L14
  constraint perpendicular L13 L15
  constraint horizontal L16
  constraint vertical L17
  constraint horizontal L18
  constraint vertical L19
  constraint midpoint L596 L598.start
  constraint perpendicular L596 L598
  constraint perpendicular L597 L599
  constraint perpendicular L599 L600
  constraint horizontal L601
  constraint vertical L602
  constraint horizontal L603
  constraint vertical L604
  constraint perpendicular L600 L605
  constraint perpendicular L596 L606
  constraint horizontal L607
  constraint vertical L608
  constraint horizontal L609
  constraint vertical L610
  measures "d25" distance of L8.start L8.end
  measures "d26" distance of L8.end L9.end
  measures "d27" distance of L9.end L10.end
  measures "d28" distance of L9.end L12.end
  measures "d29" distance of L9.end L14.end
  measures "d30" distance of L14.end L15.end
  measures "d31" distance of L15.end L16.end
  measures "d32" distance of L15.end L18.end
  measures "d37" distance of L598.end L599.end
  measures "d38" distance of L599.end L600.end
  measures "d39" distance of L600.end L601.end
  measures "d40" distance of L600.end L603.end
  measures "d41" distance of L600.end L605.end
  measures "d42" distance of L605.end L606.end
  measures "d43" distance of L606.end L607.end
  measures "d44" distance of L606.end L609.end
extrude "Extrude3" cut sketch "Sketch2" against normal blind 4 contours L7 L260 L261 L264 L266 | L7 L261 L263 L264 L265 L266 L267 | L7 L248 L249 L252 L254 | L7 L249 L251 L252 L253 L254 L255 | A26 L236 L240 | A20 L214 L216 L219 | L4 L200 L201 L204 L206 | L4 L201 L203 L204 L205 L206 L207 | L4 L188 L189 L192 L194 | L4 L189 L191 L192 L193 L194 L195 | L8 L13 L16 L18 | L8 L11 L16 L18 | L11 L12 L13 L18 | L8 L9 L10 L13 L14 L16 | L8 L10 L11 L16 | L11 L16 L17 L18 | L13 L15 L16 L18 L19 | L56 L57 L60 L62 | L56 L60 L66 L67 | L56 L60 L62 L67 | L57 L59 L60 L61 L62 L63 | L56 L63 L65 L67 | L60 L62 L63 L67 | L58 L60 L63 L64 L67 | L140 L141 L144 L146 | L140 L144 L150 L151 | L140 L144 L146 L151 | L141 L143 L144 L145 L146 L147 | L140 L147 L149 L151 | L144 L146 L147 L151 | L142 L144 L147 L148 L151 | L224 L225 L228 L230 | L224 L228 L234 L235 | L224 L228 L230 L235 | L225 L227 L228 L229 L230 L231 | L224 L231 L233 L235 | L228 L230 L231 L235 | L226 L228 L231 L232 L235 | L272 L273 L276 L278 | L272 L276 L282 L283 | L272 L276 L278 L283 | L273 L275 L276 L277 L278 L279 | L272 L279 L281 L283 | L276 L278 L279 L283 | L274 L276 L279 L280 L283 | L284 L285 L288 L290 | L284 L288 L294 L295 | L284 L288 L290 L295 | L285 L287 L288 L289 L290 L291 | L284 L291 L293 L295 | L288 L290 L291 L295 | L286 L288 L291 L292 L295 | L296 L297 L300 L302 | L296 L300 L306 L307 | L296 L300 L302 L307 | L297 L299 L300 L301 L302 L303 | L296 L303 L305 L307 | L300 L302 L303 L307 | L298 L300 L303 L304 L307 | L308 L309 L312 L314 | L308 L312 L318 L319 | L308 L312 L314 L319 | L309 L311 L312 L313 L314 L315 | L308 L315 L317 L319 | L312 L314 L315 L319 | L310 L312 L315 L316 L319 | L320 L321 L324 L326 | L320 L324 L330 L331 | L320 L324 L326 L331 | L321 L323 L324 L325 L326 L327 | L320 L327 L329 L331 | L324 L326 L327 L331 | L322 L324 L327 L328 L331 | L332 L333 L336 L338 | L332 L336 L342 L343 | L332 L336 L338 L343 | L333 L335 L336 L337 L338 L339 | L332 L339 L341 L343 | L336 L338 L339 L343 | L334 L336 L339 L340 L343 | L380 L381 L384 L386 | L380 L384 L390 L391 | L380 L384 L386 L391 | L381 L383 L384 L385 L386 L387 | L380 L387 L389 L391 | L384 L386 L387 L391 | L382 L384 L387 L388 L391 | L464 L465 L468 L470 | L464 L468 L474 L475 | L464 L468 L470 L475 | L465 L467 L468 L469 L470 L471 | L464 L471 L473 L475 | L468 L470 L471 L475 | L466 L468 L471 L472 L475 | L548 L549 L552 L554 | L548 L552 L558 L559 | L548 L552 L554 L559 | L549 L551 L552 L553 L554 L555 | L548 L555 L557 L559 | L552 L554 L555 L559 | L550 L552 L555 L556 L559 | L596 L598 L604 L606 L607 L609 | L598 L599 L604 L607 L609 | L598 L602 L603 L604 L609 | L599 L600 L601 L604 L605 L607 | L599 L602 L607 L609 | L599 L601 L602 L607 | L602 L607 L608 L609 | L611 L612 L615 L616 L617 L623 | L613 L614 L617 L618 L622 L623 | L612 L614 L615 L617 L623 | L612 L614 L617 L620 | L614 L617 L620 L622 | L612 L615 L619 L620 L623 | L612 L617 L620 L621 | L624 L625 L628 L629 L630 L636 | L626 L627 L630 L631 L635 L636 | L625 L627 L628 L630 L636 | L625 L627 L630 L633 | L627 L630 L633 L635 | L625 L628 L632 L633 L636 | L625 L630 L633 L634 | L637 L638 L641 L642 L643 L649 | L639 L640 L643 L644 L648 L649 | L638 L640 L641 L643 L649 | L638 L640 L643 L646 | L640 L643 L646 L648 | L638 L641 L645 L646 L649 | L638 L643 L646 L647